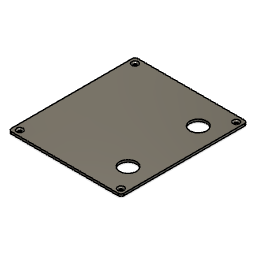
PageTurner_Lid (Autodesk Fusion 360 design; units mm, degrees)
Autodesk Fusion 360 part; units mm, degrees
sketch "Skizze1" plane through (0, 0, 0) normal (0, 1, 0) x (1, 0, 0)
  line L0 (-39.9994, 44.9914) -> (40.0006, 44.9914)
  line L1 (40.0006, 44.9914) -> (40.0006, -45.0086)
  line L2 (40.0006, -45.0086) -> (-39.9994, -45.0086)
  line L3 (-39.9994, -45.0086) -> (-39.9994, 44.9914)
  circle A0 centre (-35.9994, 40.9914) radius 1.25
  circle A1 centre (36.0006, 40.9914) radius 1.25
  circle A2 centre (36.0006, -41.0086) radius 1.25
  circle A3 centre (-35.9994, -41.0086) radius 1.25
  circle A4 centre (25.0006, 24.9914) radius 6
  circle A5 centre (25.0006, -25.0086) radius 6
  dimension "d1" = 80
  dimension "d2" = 90
  dimension "d3" = 2.5
  dimension "d4" = 4
  dimension "d5" = 4
  dimension "d6" = 2.5
  dimension "d7" = 4
  dimension "d8" = 4
  dimension "d9" = 2.5
  dimension "d10" = 4
  dimension "d11" = 4
  dimension "d12" = 2.5
  dimension "d13" = 4
  dimension "d14" = 4
  dimension "d39" = 12
  dimension "d40" = 12
  dimension "d41" = 15
  dimension "d42" = 20
  dimension "d43" = 15
  dimension "d44" = 20
  constraint horizontal L0
  constraint vertical L1
  constraint horizontal L2
  constraint vertical L3
  measures "d1" distance of L0.start L0.end
  measures "d2" distance of L0.start L2.end
  measures "d3" diameter of A3
  measures "d4" vertical distance of L2.end A3.centre
  measures "d5" horizontal distance of L2.end A3.centre
  measures "d6" diameter of A2
  measures "d7" distance of L2 A2.centre
  measures "d8" distance of L1 A2.centre
  measures "d9" diameter of A1
  measures "d10" distance of L0 A1.centre
  measures "d11" distance of L1 A1.centre
  measures "d12" diameter of A0
  measures "d13" distance of L3 A0.centre
  measures "d14" distance of L0 A0.centre
  measures "d39" diameter of A4
  measures "d40" diameter of A5
  measures "d41" distance of L1 A4.centre
  measures "d42" distance of L0 A4.centre
  measures "d43" distance of L1 A5.centre
  measures "d44" distance of L2 A5.centre
extrude "Extrusion1" add sketch "Skizze1" along normal blind 1.5
fillet "Abrundung1" radius 2 1 edges at (-39.9994, 0.75, 45.0086)
fillet "Abrundung1" radius 2 1 edges at (40.0006, 0.75, 45.0086)
fillet "Abrundung1" radius 2 1 edges at (-39.9994, 0.75, -44.9914)
fillet "Abrundung1" radius 2 1 edges at (40.0006, 0.75, -44.9914)
chamfer "Fase1" distance 1 angle 45 1 edges at (-37.1648, 1.5, -41.4434)
chamfer "Fase1" distance 1 angle 45 1 edges at (34.8352, 1.5, -41.4434)
chamfer "Fase1" distance 1 angle 45 1 edges at (-37.1648, 1.5, 40.5566)
chamfer "Fase1" distance 1 angle 45 1 edges at (34.8352, 1.5, 40.5566)
sketch "Skizze3" plane through (0, 0, 0) normal (0, -1, 0) x (1, 0, 0)
  arc A0 (38.0006, -44.9914) -> (40.0006, -42.9914) centre (38.0006, -42.9914) ccw
  line L0 (40.0006, -42.9914) -> (40.0006, 43.0086)
  arc A1 (40.0006, 43.0086) -> (38.0006, 45.0086) centre (38.0006, 43.0086) ccw
  line L1 (38.0006, 45.0086) -> (-37.9994, 45.0086)
  arc A2 (-37.9994, 45.0086) -> (-39.9994, 43.0086) centre (-37.9994, 43.0086) ccw
  line L2 (-39.9994, 43.0086) -> (-39.9994, -42.9914)
  arc A3 (-39.9994, -42.9914) -> (-37.9994, -44.9914) centre (-37.9994, -42.9914) ccw
  line L3 (-37.9994, -44.9914) -> (38.0006, -44.9914)
  circle A4 centre (-35.9994, -40.9914) radius 1.25
  circle A5 centre (36.0006, 41.0086) radius 1.25
  circle A6 centre (36.0006, -40.9914) radius 1.25
  circle A7 centre (-35.9994, 41.0086) radius 1.25
  line L4 (-36.9994, 35) -> (-34.9994, 35)
  line L5 (-34.9994, 35) -> (-34.9994, -35)
  line L6 (-34.9994, -35) -> (-36.9994, -35)
  line L7 (-36.9994, -35) -> (-36.9994, 35)
  line L8 (-30, 42.0086) -> (30, 42.0086)
  line L9 (30, 42.0086) -> (30, 40.0086)
  line L10 (30, 40.0086) -> (-30, 40.0086)
  line L11 (-30, 40.0086) -> (-30, 42.0086)
  line L12 (37.0006, 35) -> (35.0006, 35)
  line L13 (35.0006, 35) -> (35.0006, -35)
  line L14 (35.0006, -35) -> (37.0006, -35)
  line L15 (37.0006, -35) -> (37.0006, 35)
  line L16 (30, -41.9914) -> (-30, -41.9914)
  line L17 (-30, -41.9914) -> (-30, -39.9914)
  line L18 (-30, -39.9914) -> (30, -39.9914)
  line L19 (30, -39.9914) -> (30, -41.9914)
  circle A8 centre (25.0006, -24.9914) radius 6
  circle A9 centre (25.0006, 25.0086) radius 6
  dimension "d29" = 2
  dimension "d30" = 2
  dimension "d31" = 2
  dimension "d32" = 2
  dimension "d33" = 3
  dimension "d34" = 3
  dimension "d35" = 3
  dimension "d36" = 3
  constraint horizontal L4
  constraint vertical L5
  constraint horizontal L6
  constraint vertical L7
  constraint horizontal L8
  constraint vertical L9
  constraint horizontal L10
  constraint vertical L11
  constraint horizontal L12
  constraint vertical L13
  constraint horizontal L14
  constraint vertical L15
  constraint horizontal L16
  constraint vertical L17
  constraint horizontal L18
  constraint vertical L19
  measures "d29" distance of L16.start L18.end
  measures "d30" distance of L13.end L14.end
  measures "d31" distance of L5.end L6.end
  measures "d32" distance of L8.start L10.end
  measures "d33" distance of L2 L4.start
  measures "d34" distance of L1 L8.start
  measures "d35" distance of L0 L12.start
  measures "d36" distance of L3 L16.start
extrude "Extrusion2" add sketch "Skizze3" along normal blind 1 contours L4 L5 L6 L7 | L8 L9 L10 L11 | L12 L13 L14 L15 | L16 L17 L18 L19
